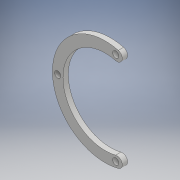
# Autodesk Inventor part: Reverse Lever Ring
Saved by Autodesk Inventor 2017 (Build 210142000, 142)
## iProperties
Created: 2018-11-20
Part Number: Reverse Lever Ring
Material: Generic
Document SubType Name: Modeling
Designer: Arman Grewal
Density: 1 g/cm^3
Appearance: Default
Author: Arman Grewal
Autodesk Inventor part; units mm, degrees
ref_plane "YZ Plane" through (0, 0, 0) normal (1, 0, 0) x (0, 1, 0)
ref_plane "XZ Plane" through (0, 0, 0) normal (0, 1, 0) x (-1, 0, 0)
ref_plane "XY Plane" through (0, 0, 0) normal (0, 0, 1) x (1, 0, 0)
sketch "Sketch1" plane through (0, 0, 0) normal (0, 1, 0) x (-1, 0, 0)
  arc A0 (-10.5785, -28.0731) -> (-10.5785, 28.0731) centre (0, 0) ccw
  arc A1 (-23.5162, 13.2661) -> (-10.5785, 24.8414) centre (0, 0) ccw construction
  arc A2 (-10.5785, -21.5429) -> (-10.5785, 21.5429) centre (0, 0) ccw
  circle A3 centre (27, 0) radius 1.75
  circle A4 centre (16.8342, 21.1095) radius 1.75
  circle A5 centre (-6.0081, 26.3231) radius 1.75
  circle A6 centre (-24.3262, 11.7149) radius 1.75
  circle A7 centre (-24.3262, -11.7149) radius 1.75
  circle A8 centre (-6.0081, -26.3231) radius 1.75
  circle A9 centre (16.8342, -21.1095) radius 1.75
  line L0 (-10.5785, 28.0731) -> (-8.5262, 22.4344)
  line L1 (-10.5785, 28.0731) -> (-4.578, 28.0731) construction
  line L2 (-10.5785, -28.0731) -> (-8.5262, -22.4344)
  dimension "d2" = 60
  dimension "d3" = 54
  dimension "d4" = 48
  dimension "d5" = 3.5
  dimension "d6" = 360
  dimension "d7" = 70
  constraints: 9 centre point, 9 point on circle, 6 end point, 3 coincident, 1 equal length, 1 horizontal, 1 tangent, 18 other
  measures "d2" diameter of A0
  measures "d3" diameter of A1
  measures "d4" diameter of A2
  measures "d5" diameter of A3
  measures "d7" angle of L0 L1
extrude "Extrusion1" add sketch "Sketch1" along normal blind 3 contours L2 A2 L0 A0 | A4 | A9
fillet "Fillet1" radius 3 4 edges at (10.5785, 1.5, 28.0731) (8.5262, 1.5, 22.4344) (8.5262, 1.5, -22.4344) (10.5785, 1.5, -28.0731)
body "Solid1"
